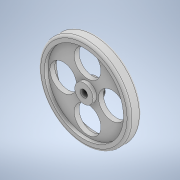
# Autodesk Inventor part: fly_wheel
Saved by Autodesk Inventor 2022.2 (Build 262287010, 287A)
## iProperties
Created: 2022-05-04
Part Number: fly_wheel
Material: Genérico
Document SubType Name: Modeling
Designer: 19710060
Density: 1 g/cm^3
Appearance: Padrão
Author: 19710060
Autodesk Inventor part; units mm, degrees
ref_plane "XZ Plane" through (0, 0, 0) normal (0, 1, 0) x (-1, 0, 0)
ref_plane "XY Plane" through (0, 0, 0) normal (0, 0, 1) x (1, 0, 0)
sketch "Esboço1" plane through (0, 0, 0) normal (0, 0, 1) x (1, 0, 0)
  circle A0 centre (0, 0) radius 37.5
  circle A1 centre (0, 0) radius 32.5
  circle A2 centre (0, 0) radius 20
  circle A3 centre (20, 0) radius 11
  circle A4 centre (0, 20) radius 11
  circle A5 centre (-20, 0) radius 11
  circle A6 centre (0, -20) radius 11
  circle A7 centre (0, 0) radius 7.5
  circle A8 centre (0, 0) radius 3
  dimension "d2" = 40
  dimension "d17" = 1
  dimension "d0" = 75
  dimension "d1" = 65
  dimension "d3" = 22
  dimension "d6" = 360
  dimension "d8" = 15
  dimension "d9" = 6
  constraints: 8 centre point, 5 coincident, 1 horizontal alignment, 11 other
  measures "d0" diameter of A0
  measures "d1" diameter of A1
  measures "d3" diameter of A3
  measures "d8" diameter of A7
  measures "d9" diameter of A8
extrude "Extrusão1" add sketch "Esboço1" along normal mid plane 10 contours A0
extrude "Extrusão2" add sketch "Esboço1" along normal mid plane 4 contours A1 | A3 A2 A6 A5 A4
extrude "Extrusão3" add sketch "Esboço1" along normal mid plane 10 contours A7
fillet "Arredondamento1" radius 2 2 edges at (-37.5, 0, 5) (-37.5, 0, -5)
fillet "Arredondamento2" [suppressed]
sketch "Esboço2" plane through (0, 0, 2) normal (0, 0, 1) x (1, 0, 0)
  point P0 (0, 0)
  dimension "d17" = 1
ref_plane "Work Plane3" through (7.5, 0, 0) normal (1, 0, 0) x (0, 1, 0)
sketch "Sketch8" plane through (7.5, 0, 0) normal (1, 0, 0) x (0, 1, 0)
  line L0 (-7.5, -5) -> (7.5, -5) projected
  line L1 (7.5, -2) -> (-7.5, -2) projected
  line L2 (0, -2) -> (0, -4.5)
  circle A0 centre (0, -3.25) radius 1.25
  point P0 (0, 0)
  dimension "d17" = 1
  dimension "d34" = 2.5
  constraints: 2 end point, 2 midpoint, 1 vertical, 1 vertical alignment, 2 other
  measures "d34" distance of L2.start L2.end
sketch "Sketch9" plane through (0, 0, 0) normal (0, 1, 0) x (-1, 0, 0)
  line L0 (-3.4847, 0.1554) -> (-11.509, -4.1521)
  line L1 (-3, 5) -> (-3, -5) projected
  line L2 (-2.8935, -0.9459) -> (-10.9178, -5.2534)
  line L3 (-10.9178, -5.2534) -> (-11.509, -4.1521)
  line L4 (-3.4847, 0.1554) -> (-2.8935, -0.9459)
  point P0 (0, 0)
  point P1 (-7.5, -2)
  point P2 (-3, -1.0031)
  point P3 (-3, -0.7476)
  dimension "d40" = 1.25
  constraints: 8 end point, 2 parallel, 1 point on line
  measures "d40" distance between parallel lines of L0 L2
revolve "Revolution1" cut sketch "Sketch9" angle 360 about axis through (2.8935, 0, -0.9459) along (0.8810792, 0, -0.4729688) contours L4 L1 L2 L3 L0
